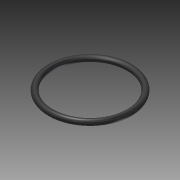
# Autodesk Inventor part: oringlarge
Saved by Autodesk Inventor 2015 (Build 190159000, 159)
## iProperties
Created: 2015-02-17
Part Number: oringlarge
Material: Rubber, Silicone
Document SubType Name: Modeling
Designer: Hanjie
Density: 1.25 g/cm^3
Appearance: Rubber - Black - Version 1.1
Author: Hanjie
Autodesk Inventor part; units mm, degrees
ref_plane "YZ Plane" through (0, 0, 0) normal (1, 0, 0) x (0, 1, 0)
ref_plane "XZ Plane" through (0, 0, 0) normal (0, 1, 0) x (-1, 0, 0)
ref_plane "XY Plane" through (0, 0, 0) normal (0, 0, 1) x (1, 0, 0)
sketch "Sketch1" plane through (0, 0, 0) normal (0, 0, 1) x (1, 0, 0)
  line L0 (0, 0) -> (35.56, 0)
  circle A0 centre (35.56, 0) radius 2.54
  line L1 (0, -3.556) -> (0, 3.556) projected
  dimension "d0" = 35.56
  dimension "d1" = 5.08
  constraints: 2 end point, 1 centre point, 1 coincident, 1 horizontal
  measures "d0" distance of L0.start L0.end
  measures "d1" diameter of A0
revolve "Revolution1" add sketch "Sketch1" angle 360 about axis through (0, -10, 0) along (0, 1, 0)
body "Solid1"
